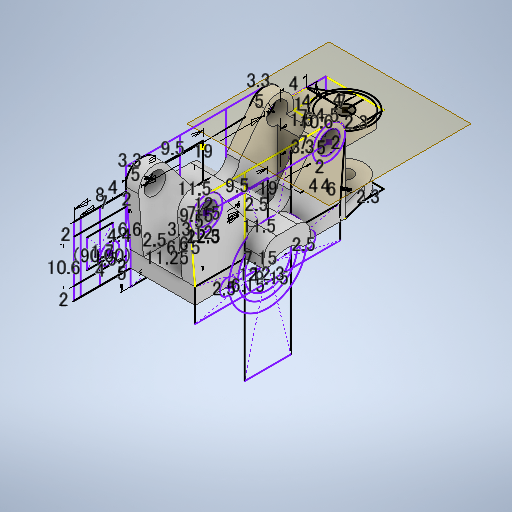
# Autodesk Inventor part: ikafly5.3d
Saved by Autodesk Inventor 2025 (Build 290162000, 162)
## iProperties
Created: 2024-06-20
Part Number: ikafly5.3d
Material: 一般
Document SubType Name: Modeling
Designer: Saigusa
Density: 1 g/cm^3
Appearance: 既定
Author: Saigusa
Autodesk Inventor part; units mm, degrees
ref_plane "YZ Plane" through (0, 0, 0) normal (1, 0, 0) x (0, 1, 0)
ref_plane "XZ Plane" through (0, 0, 0) normal (0, 1, 0) x (-1, 0, 0)
ref_plane "XY Plane" through (0, 0, 0) normal (0, 0, 1) x (1, 0, 0)
sketch "スケッチ1" plane through (0, 0, 0) normal (1, 0, 0) x (0, 1, 0)
  circle A0 centre (0, 0) radius 4.575
  circle A1 centre (0, 0) radius 3.575
  line L0 (0, 0) -> (0, 6)
  line L1 (0, 6) -> (0, -6)
  line L2 (0, 0) -> (11.5, 0)
  line L3 (11.5, 0) -> (11.5, 9.5)
  line L4 (11.5, 9.5) -> (11.5, -9.5)
  circle A2 centre (11.5, 9.5) radius 1.65
  circle A3 centre (11.5, -9.5) radius 1.65
  line L5 (0, 0) -> (0, 11.25)
  line L6 (0, 11.25) -> (0, -11.25)
  line L7 (-2.5, -11.25) -> (2.5, -11.25)
  line L8 (2.5, -11.25) -> (2.5, 11.25)
  line L9 (2.5, 11.25) -> (-2.5, 11.25)
  line L10 (-2.5, 11.25) -> (-2.5, -11.25)
  line L11 (-2.5, -11.25) -> (2.5, 11.25) construction
  line L12 (2.5, -11.25) -> (-2.5, 11.25) construction
  circle A4 centre (11.5, 9.5) radius 2.5
  circle A5 centre (11.5, -9.5) radius 2.5
  line L13 (2.5, 11.25) -> (11.2899, 11.9912)
  line L14 (2.5, -11.25) -> (11.2899, -11.9912)
  line L15 (14, 9.5) -> (14, -9.5)
  line L16 (0, -3.575) -> (14, -3.575)
  line L17 (0, 3.575) -> (14, 3.575)
  circle A6 centre (0, 0) radius 6
  line L18 (0, 0) -> (0, 6.15)
  line L19 (0, 6.15) -> (0, -6.15)
  circle A7 centre (0, 6.15) radius 1.25
  circle A8 centre (0, -6.15) radius 1.25
  line L20 (11.5, 9.5) -> (9, 9.5)
  line L21 (9, 9.5) -> (0, 9.5)
  line L22 (11.5, 9.5) -> (14, 9.5)
  line L23 (14, 9.5) -> (14, 11.9912)
  line L24 (14, 11.9912) -> (11.5, 11.9912)
  line L25 (11.5, 11.9912) -> (11.5, 9.5)
  line L26 (11.5, 11.9912) -> (0, 11.9912)
  line L27 (0, 11.9912) -> (0, 11.25)
  line L28 (0, 11.9912) -> (2, 11.9912)
  line L29 (2, 11.9912) -> (8.6, 11.9912)
  line L30 (8.6, 11.9912) -> (10.6, 11.9912)
  line L31 (0, 11.9912) -> (10.6, 11.9912)
  line L32 (10.6, 11.9912) -> (10.6, 19.9912)
  line L33 (10.6, 19.9912) -> (0, 19.9912)
  line L34 (0, 19.9912) -> (0, 11.9912)
  line L35 (0, 11.9912) -> (10.6, 11.9912)
  line L36 (10.6, 11.9912) -> (10.6, 15.9912)
  line L37 (10.6, 15.9912) -> (0, 15.9912)
  line L38 (0, 15.9912) -> (0, 11.9912)
  line L39 (0, 11.9912) -> (2, 11.9912)
  line L40 (2, 11.9912) -> (2, 19.9912)
  line L41 (2, 19.9912) -> (0, 19.9912)
  line L42 (0, 19.9912) -> (0, 11.9912)
  line L43 (10.6, 11.9912) -> (8.6, 11.9912)
  line L44 (8.6, 11.9912) -> (8.6, 19.9912)
  line L45 (8.6, 19.9912) -> (10.6, 19.9912)
  line L46 (10.6, 19.9912) -> (10.6, 11.9912)
  line L47 (0, 11.9912) -> (10.6, 11.9912)
  line L48 (10.6, 11.9912) -> (10.6, 18.9912)
  line L49 (10.6, 18.9912) -> (0, 18.9912)
  line L50 (0, 18.9912) -> (0, 11.9912)
  line L51 (0, 15.9912) -> (5.3, 15.9912)
  line L52 (7.5, 17.9912) -> (3.1, 17.9912)
  line L53 (3.1, 17.9912) -> (3.1, 13.9912)
  line L54 (3.1, 13.9912) -> (7.5, 13.9912)
  line L55 (7.5, 13.9912) -> (7.5, 17.9912)
  line L56 (7.5, 17.9912) -> (3.1, 13.9912) construction
  line L57 (3.1, 17.9912) -> (7.5, 13.9912) construction
  line L58 (5.3, 15.9912) -> (3.6, 15.9912)
  line L59 (3.6, 15.9912) -> (3.6, 14.4912)
  line L60 (3.6, 15.9912) -> (5.1, 15.9912) construction
  circle A9 centre (3.6, 14.4912) radius 0.5
  circle A10 centre (3.6, 14.4912) radius 1.5
  line L61 (5.1, 14.4912) -> (5.1, 11.9912)
  line L62 (11.5, -9.5) -> (0, -9.5)
  line L63 (0, -9.5) -> (0, -11.9912)
  line L64 (0, -11.9912) -> (11.5, -11.9912)
  line L65 (11.5, -11.9912) -> (11.5, -9.5)
  line L66 (0, -11.9912) -> (2, -11.9912)
  line L67 (2, -11.9912) -> (2, -18.9912)
  line L68 (2, -18.9912) -> (0, -18.9912)
  line L69 (0, -18.9912) -> (0, -11.9912)
  line L70 (0, -11.9912) -> (10.6, -11.9912)
  line L71 (10.6, -11.9912) -> (10.6, -15.9912)
  line L72 (10.6, -15.9912) -> (0, -15.9912)
  line L73 (0, -15.9912) -> (0, -11.9912)
  line L74 (10.6, -11.9912) -> (8.6, -11.9912)
  line L75 (8.6, -11.9912) -> (8.6, -18.9912)
  line L76 (8.6, -18.9912) -> (10.6, -18.9912)
  line L77 (10.6, -18.9912) -> (10.6, -11.9912)
  line L78 (2, -15.9912) -> (5.3, -15.9912)
  line L79 (3.05, -13.9912) -> (7.55, -13.9912)
  line L80 (7.55, -13.9912) -> (7.55, -17.9912)
  line L81 (7.55, -17.9912) -> (3.05, -17.9912)
  line L82 (3.05, -17.9912) -> (3.05, -13.9912)
  line L83 (3.05, -13.9912) -> (7.55, -17.9912) construction
  line L84 (7.55, -13.9912) -> (3.05, -17.9912) construction
  line L85 (5.3, -15.9912) -> (7, -15.9912)
  line L86 (7, -15.9912) -> (6.9874, -14.4912)
  circle A11 centre (6.9874, -14.4912) radius 0.5
  circle A12 centre (6.9874, -14.4912) radius 1.5
  line L87 (6.9874, -14.4912) -> (5.4874, -14.4912)
  line L88 (5.4874, -14.4912) -> (5.4874, -11.9912)
  line L89 (10.6, -11.9912) -> (10.6, -9.5)
  point P0 (0, 4.575)
  point P1 (0, -4.575)
  point P2 (2.5, 3.575)
  point P3 (2.5, 2.5555)
  point P4 (2.5, -2.5555)
  point P5 (2.5, -3.575)
  point P6 (0, 7.4)
  point P7 (0, 4.9)
  point P8 (0, -4.9)
  point P9 (0, -7.4)
  point P10 (2.5, 5.4544)
  point P11 (2.5, -5.4544)
  point P12 (4.8186, 3.575)
  point P13 (4.8186, -3.575)
  point P14 (2.8548, 3.575)
  point P15 (2.8548, -3.575)
  point P16 (9.85, 9.5)
  point P17 (11.5, 11.15)
  point P18 (11.5, -11.15)
  point P19 (9.85, -9.5)
  point P20 (5.5732, -13.9912)
  point P21 (6.9749, -15.9912)
  point P22 (8.6, -15.9912)
  point P23 (5.4874, -13.9912)
  point P24 (10.6, -10.8829)
  dimension "d0" = 9.15
  dimension "d1" = 7.15
  dimension "d2" = 6
  dimension "d3" = 12
  dimension "d6" = 11.5
  dimension "d7" = 9.5
  dimension "d8" = 19
  dimension "d9" = 3.3
  dimension "d10" = 3.3
  dimension "d11" = 11.25
  dimension "d12" = 22.5
  dimension "d13" = 5
  dimension "d14" = 5
  dimension "d15" = 5
  dimension "d28" = 12
  dimension "d29" = 6.15
  dimension "d30" = 12.3
  dimension "d31" = 2.5
  dimension "d32" = 2.5
  dimension "d99" = 2
  dimension "d100" = 6.6
  dimension "d101" = 2
  dimension "d114" = 10.6
  dimension "d115" = 8
  dimension "d116" = 4
  dimension "d117" = 2
  dimension "d118" = 2
  dimension "d119" = 7
  dimension "d120" = 4.4
  dimension "d121" = 4
  dimension "d122" = 1.7
  dimension "d123" = 1.5
  dimension "d124" = 90
  dimension "d125" = 2
  dimension "d126" = 7
  dimension "d127" = 10.6
  dimension "d128" = 4
  dimension "d129" = 7
  dimension "d130" = 4.5
  dimension "d131" = 4
  dimension "d132" = 1.5
  dimension "d133" = 1
  constraints: 180 end point, 27 parallel, 26 point on line, 21 perpendicular, 17 horizontal, 13 coincident, 12 centre point, 9 midpoint, 9 point on circle, 7 tangent, 2 vertical, 1 horizontal alignment, 2 other
  measures "d0" diameter of A0
  measures "d1" diameter of A1
  measures "d2" distance of L0.start L0.end
  measures "d3" distance of L0.end L1.end
  measures "d6" distance of L0.start L2.end
  measures "d7" distance of L2.end L3.end
  measures "d8" distance of L3.end L4.end
  measures "d9" diameter of A2
  measures "d10" diameter of A3
  measures "d11" distance of L0.start L5.end
  measures "d12" distance of L5.end L6.end
  measures "d13" distance of L9.end L8.end
  measures "d14" diameter of A4
  measures "d15" diameter of A5
  measures "d28" diameter of A6
  measures "d29" distance of L18.start L18.end
  measures "d30" distance of L18.end L19.end
  measures "d31" diameter of A7
  measures "d32" diameter of A8
  measures "d99" distance of L26.end L28.end
  measures "d100" distance of L28.end L29.end
  measures "d101" distance of L29.end L30.end
  measures "d114" distance of L33.end L32.end
  measures "d115" distance of L32.end L31.end
  measures "d116" distance of L36.end L35.end
  measures "d117" distance of L41.end L40.end
  measures "d118" distance of L44.end L45.end
  measures "d119" distance of L48.end L47.end
  measures "d120" distance of L54.end L53.end
  measures "d121" distance of L53.end L52.end
  measures "d122" distance of L51.end L58.end
  measures "d123" distance of L58.end L59.end
  measures "d124" angle of L59 L60
  measures "d125" distance of L67.end L68.end
  measures "d126" distance of L66.end L67.end
  measures "d127" distance of L71.end L72.end
  measures "d128" distance of L70.end L71.end
  measures "d129" distance of L75.end L74.end
  measures "d130" distance of L80.end L81.end
  measures "d131" distance of L79.end L80.end
  measures "d132" distance of L85.end L86.end
  measures "d133" diameter of A11
extrude "押し出し7" add sketch "スケッチ1" along normal blind 2 contours L2 A6 L16 A0 | A0 L17 A6 L2 | A0 L8 A6 L17 | L16 A6 L8 A0 | A6 L17 L3 L2 | L2 L4 L16 A6 | A0 L0 A7 A6 L8 | A6 L8 L21 A4 L3 L17 | L8 A6 A8 L1 A0 | L16 L4 A5 L62 L8 A6 | L3 L17 L15 L16 L4 | A6 A7 L5 L21 L8 | L3 A4 L15 L17 | L8 L62 L6 A8 A6 | L16 L15 A5 L4 | L21 L5 L9 L8 | L8 L13 A4 L21 | A4 L20 A2 L3 | L3 A2 L22 A4 | L62 A5 L89 L14 L8 | L8 L7 L6 L62 | A5 L64 L65 A3 L4 | L4 A3 L62 A5 | A4 L26 L25 A2 L20 | L22 A2 L25 L24 A4 | L62 A3 L89 A5 | A4 L24 L26 | L89 A5 L14 | L89 A3 L65 L64 A5
extrude "押し出し8" add sketch "スケッチ1" along normal blind 10 contours L2 A6 L16 A0 | A0 L17 A6 L2 | A0 L8 A6 L17 | L16 A6 L8 A0 | A6 L17 L3 L2 | L2 L4 L16 A6 | A0 L0 A7 A6 L8 | L8 A6 A8 L1 A0 | L3 L17 L15 L16 L4 | A6 A7 L5 L21 L8 | L8 L62 L6 A8 A6 | L0 A6 A7 | L21 L5 L9 L8 | A6 L5 A7 | A8 A6 L1 | L8 L7 L6 L62 | A8 L6 A6 picked at (0.2292, 5.6392) picked at (0.3961, 6.4211) picked at (0.2292, -5.6392) picked at (0.3961, -6.4211)
sketch "スケッチ6" plane through (10, 0, 0) normal (1, 0, 0) x (0, 0, -1)
  line L0 (0, 0) -> (-6.15, 0)
  line L1 (-6.15, 0) -> (6.15, 0)
  circle A0 centre (-6.15, 0) radius 1.25
  circle A1 centre (6.15, 0) radius 1.25
  line L2 (-11.25, 2.5) -> (11.25, 2.5)
  line L3 (11.25, 2.5) -> (11.25, -2.5)
  line L4 (11.25, -2.5) -> (-11.25, -2.5)
  line L5 (-11.25, -2.5) -> (-11.25, 2.5)
  line L6 (-11.25, 2.5) -> (11.25, -2.5) construction
  line L7 (11.25, 2.5) -> (-11.25, -2.5) construction
  line L8 (0, 0) -> (0, 11.5)
  line L9 (0, 11.5) -> (-9.5, 11.5)
  line L10 (-9.5, 11.5) -> (9.5, 11.5)
  circle A2 centre (-9.5, 11.5) radius 1.65
  circle A3 centre (-9.5, 11.5) radius 2.5
  circle A4 centre (9.5, 11.5) radius 1.65
  circle A5 centre (9.5, 11.5) radius 2.5
  circle A6 centre (0, 0) radius 6
  circle A7 centre (0, 0) radius 4.575
  arc A8 (11.9912, 11.2899) -> (9.5, 14) centre (9.5, 11.5) ccw projected
  line L11 (11.25, 2.5) -> (11.9912, 11.2899)
  line L12 (-11.9912, 11.2899) -> (-11.25, 2.5) projected
  line L13 (-11.25, 2.5) -> (-11.9912, 11.2899)
  line L14 (9.5, 14) -> (-9.5, 14) projected
  arc A9 (-9.5, 14) -> (-11.9912, 11.2899) centre (-9.5, 11.5) ccw projected
  line L15 (-9.5, 14) -> (9.5, 14)
  circle A10 centre (0, 0) radius 3.575
  line L16 (-3.575, 14) -> (-3.575, 4.8186) projected
  line L17 (3.575, -14) -> (-3.575, -14)
  line L18 (-3.575, -14) -> (-3.575, 14)
  line L19 (-3.575, 14) -> (3.575, 14)
  line L20 (3.575, 14) -> (3.575, -14)
  line L21 (3.575, -14) -> (-3.575, 14) construction
  line L22 (-3.575, -14) -> (3.575, 14) construction
  point P0 (-5.4544, 2.5)
  point P1 (5.4544, 2.5)
  point P2 (7, 11.5)
  point P3 (-7, 11.5)
  point P4 (-3.575, 11.5)
  point P5 (-3.575, 4.8186)
  point P6 (-3.575, 2.5)
  point P7 (-2.5555, 2.5)
  point P8 (2.5555, 2.5)
  point P9 (3.575, 2.5)
  point P10 (3.575, 11.5)
  dimension "d69" = 12
  dimension "d56" = 6.15
  dimension "d57" = 12.3
  dimension "d58" = 2.5
  dimension "d59" = 2.5
  dimension "d62" = 11.5
  dimension "d63" = 9.5
  dimension "d64" = 19
  dimension "d65" = 3.3
  dimension "d66" = 5
  dimension "d67" = 3.3
  dimension "d68" = 5
  dimension "d70" = 9.15
  dimension "d79" = 7.15
  constraints: 40 end point, 9 coincident, 8 centre point, 5 equal length, 4 horizontal, 4 midpoint, 3 perpendicular, 2 point on line, 2 tangent, 1 vertical, 2 other
  measures "d56" distance of L0.start L0.end
  measures "d57" distance of L0.end L1.end
  measures "d58" diameter of A0
  measures "d59" diameter of A1
  measures "d62" distance of L0.start L8.end
  measures "d63" distance of L8.end L9.end
  measures "d64" distance of L9.end L10.end
  measures "d65" diameter of A2
  measures "d66" diameter of A3
  measures "d67" diameter of A4
  measures "d68" diameter of A5
  measures "d70" diameter of A7
  measures "d79" diameter of A10
extrude "押し出し9" add sketch "スケッチ6" against normal blind 2 contours L2 L12 A3 L9 L16 A6 | L16 L9 L8 A6 | A6 L20 L10 A5 L11 L2 | A6 L8 L10 L20 | L16 L14 L20 L10 L9 | L9 A3 L14 L16 | L20 L14 A5 L10 | A3 | A5
extrude "押し出し10" add sketch "スケッチ1" against normal blind 0.5 contours L2 A6 L16 A0 | A0 L17 A6 L2 | A6 L17 L3 L2 | L2 L4 L16 A6 | L3 L17 L15 L16 L4
sketch "スケッチ7" plane through (-0.5, 0, 0) normal (-1, 0, 0) x (0, 0, 1)
  circle A0 centre (0, 0) radius 3.575
  line L0 (-9.5, 14) -> (9.5, 14) projected
  line L1 (-3.575, 14) -> (3.575, 14)
  circle A1 centre (0, 0) radius 4.575
  line L2 (-11.25, 0) -> (-11.25, 2.5) projected
  line L3 (11.25, -2.5) -> (-11.25, -2.5)
  line L4 (-11.25, -2.5) -> (-11.25, 2.5)
  line L5 (-11.25, 2.5) -> (11.25, 2.5)
  line L6 (11.25, 2.5) -> (11.25, -2.5)
  line L7 (11.25, -2.5) -> (-11.25, 2.5) construction
  line L8 (-11.25, -2.5) -> (11.25, 2.5) construction
  line L9 (-3.575, 14) -> (-3.575, 0)
  line L10 (3.575, 14) -> (3.575, 0)
  point P0 (-3.575, 2.5)
  point P1 (-2.5555, 2.5)
  point P2 (2.5555, 2.5)
  point P3 (3.575, 2.5)
  dimension "d75" = 7.15
  dimension "d76" = 5
  constraints: 18 end point, 2 centre point, 2 coincident, 2 midpoint, 2 parallel, 2 point on circle, 2 point on line, 2 tangent, 1 horizontal, 1 perpendicular
  measures "d75" diameter of A0
  measures "d76" distance of L3.end L2.end
extrude "押し出し11" add sketch "スケッチ7" along normal blind 3 contours A0 L5 L9 A1 L10 | A1 L9 L0 L10
extrude "押し出し12" add sketch "スケッチ6" along normal blind 3 contours L2 L18 A7 L8 A10 | A10 L8 A7 L20 L2 | L18 A6 L8 A7 | A7 L8 A6 L20 | L16 L9 L8 A6 | A6 L8 L10 L20 | L16 L14 L20 L10 L9
hole "穴1" at (0, 0, -6.15) at (0, 0, 6.15) direction (1, 0, 0) diameter 2.4 depth 3
sketch "スケッチ8" plane through (13, 0, 0) normal (1, 0, 0) x (0, 0, -1)
  line L0 (-3.575, 2.5) -> (-3.575, 14) projected
  line L1 (3.575, 14) -> (3.575, 2.5) projected
  line L2 (-3.575, 14) -> (3.575, 14)
  line L3 (3.575, 14) -> (3.575, 2.5)
  line L4 (3.575, 2.5) -> (-3.575, 2.5)
  line L5 (-3.575, 2.5) -> (-3.575, 14)
  circle A0 centre (0, 0) radius 6
  line L6 (-3.575, 14) -> (3.575, 14)
  line L7 (3.575, 14) -> (3.575, 6)
  line L8 (3.575, 6) -> (-3.575, 6)
  line L9 (-3.575, 6) -> (-3.575, 14)
  dimension "d89" = 12
  constraints: 16 end point, 4 parallel, 2 horizontal, 2 perpendicular, 1 centre point, 1 coincident, 1 point on line
  measures "d89" diameter of A0
extrude "押し出し13" cut sketch "スケッチ8" against normal blind 16.5 contours L0 L2 L1 L8
fillet "フィレット1" radius 2 10 edges at (11.5, 6, -3.575) (11.5, 6, 3.575) (9, 6, 3.575) (9, 6, -3.575) (5, 6, 3.575) (5, 6, -3.575) (1, 6, 3.575) (-1.75, 6, 3.575) (1, 6, -3.575) (-1.75, 6, -3.575)
sketch "スケッチ9" plane through (10, 0, 0) normal (1, 0, 0) x (0, 0, -1)
  arc A0 (2.5555, 2.5) -> (-2.5555, 2.5) centre (0, 0) ccw projected
  line L0 (0, 0) -> (0, 11.5)
  line L1 (0, 11.5) -> (-9.5, 11.5)
  circle A1 centre (9.5, 11.5) radius 1.65 projected
  line L2 (-9.5, 11.5) -> (9.5, 11.5)
  circle A2 centre (-9.5, 11.5) radius 2.5
  circle A3 centre (9.5, 11.5) radius 2.5
  arc A4 (-3.575, 8) -> (-1.575, 6) centre (-1.575, 8) ccw projected
  line L3 (-3.575, 8) -> (-7.5334, 13.0435)
  arc A5 (1.575, 6) -> (3.575, 8) centre (1.575, 8) ccw projected
  line L4 (3.575, 8) -> (7.5334, 13.0435)
  line L5 (9.5, 14) -> (3.575, 14) projected
  line L6 (-3.575, 8) -> (3.575, 8)
  line L7 (3.575, 8) -> (3.575, 14)
  line L8 (3.575, 14) -> (-3.575, 14)
  line L9 (-3.575, 14) -> (-3.575, 8)
  line L10 (-3.575, 8) -> (-9.5, 8)
  line L11 (-9.5, 8) -> (-9.5, 14)
  line L12 (-9.5, 14) -> (-3.575, 14)
  line L13 (-3.575, 14) -> (-3.575, 8)
  line L14 (3.575, 8) -> (9.5, 8)
  line L15 (9.5, 8) -> (9.5, 14)
  line L16 (9.5, 14) -> (3.575, 14)
  line L17 (3.575, 14) -> (3.575, 8)
  dimension "d93" = 11.5
  dimension "d94" = 9.5
  dimension "d95" = 5
  dimension "d96" = 5
  constraints: 34 end point, 6 parallel, 4 perpendicular, 3 horizontal, 3 point on circle, 2 centre point, 2 coincident, 2 tangent, 1 vertical
  measures "d93" distance of L0.start L0.end
  measures "d94" distance of L0.end L1.end
  measures "d95" diameter of A2
  measures "d96" diameter of A3
extrude "押し出し14" cut sketch "スケッチ9" against normal blind 16.5 contours L3 L1 L9 | L7 L2 L4 | L1 L3 A2 L12 L9 | L7 L5 A3 L4 L2
ref_plane "作業平面2" through (10, 14, -9.5) normal (0, 1, 0) x (-1, 0, 0)
extrude "押し出し16" add sketch "スケッチ1" along normal blind 10 contours L62 A5 L89 L14 L8 | L8 L7 L6 L62 | L14 L89 L64 L63 L7 | L62 A3 L89 A5
extrude "押し出し17" add sketch "スケッチ1" along normal blind 2 contours L75 L72 L80 A12 L79 L88 L64 | A12 L87 A11 L86 | L86 A11 L79 L80 A12 | A12 L80 L72 | L79 A12 L88 | A12 L80 L79 | L79 A11 L87 A12
extrude "押し出し18" add sketch "スケッチ1" along normal blind 9 contours L64 L67 L72 L69 | L71 L72 L75 L64 | L72 L67 L68 L69 | L77 L76 L75 L72
sketch "スケッチ11" plane through (0, 10.6, -11.9912) normal (0, 1, 0) x (1, 0, 0)
  line L0 (9, 0) -> (0, 0) projected
  line L1 (2, 4) -> (2, 0) projected
  line L2 (0, 0) -> (2, 0)
  line L3 (2, 0) -> (2, 4)
  line L4 (2, 4) -> (0, 4)
  line L5 (0, 4) -> (0, 0)
  line L6 (2, 4) -> (6, 4)
  circle A0 centre (6, 4) radius 1.15
  circle A1 centre (6, 4) radius 3.5
  circle A2 centre (6, 4) radius 4
  line L7 (6, 4) -> (6, 7)
  line L8 (0, 7) -> (9, 7) projected
  line L9 (4.85, 4) -> (4.85, 7)
  line L10 (4.85, 7) -> (0, 4)
  line L11 (0, -4.6412) -> (0, 7) projected
  line L12 (6, 4) -> (0, 4)
  line L13 (0, 4) -> (0, 7)
  line L14 (0, 7) -> (6, 7)
  line L15 (6, 7) -> (6, 4)
  line L16 (6, 4) -> (9, 4)
  line L17 (9, 4) -> (9, 7)
  line L18 (9, 7) -> (6, 7)
  line L19 (6, 7) -> (6, 4)
  point P0 (0, -11.9912)
  point P1 (9, 5.8028)
  point P2 (7.8028, 7)
  dimension "d141" = 2.3
  dimension "d140" = 4
  dimension "d142" = 7
  constraints: 32 end point, 7 parallel, 4 point on line, 3 coincident, 3 horizontal, 3 perpendicular, 2 horizontal alignment, 2 vertical, 1 centre point, 4 other
  measures "d140" distance of L1.start L6.end
  measures "d142" diameter of A1
extrude "押し出し19" cut sketch "スケッチ11" against normal blind 10.6 contours A0 L7 L6 | L6 L16 A0 | L7 A0 L16
extrude "押し出し20" cut sketch "スケッチ11" against normal blind 2 contours L11 L8 A2 L10 | A2 L8 A1 L10 | L17 A1 L8 A2 | A2 L8 L17 | A1 L8 L10
sketch "スケッチ12" plane through (0, 0, -4.575) normal (0, -1, 0) x (1, 0, 0)
  line L0 (2, -7.4162) -> (9, -7.4162) projected
  line L1 (0, -14.4162) -> (9, -14.4162) projected
  line L2 (9, -7.4162) -> (0, -7.4162)
  line L3 (0, -7.4162) -> (0, -14.4162)
  line L4 (0, -14.4162) -> (9, -14.4162)
  line L5 (9, -14.4162) -> (9, -7.4162)
  line L6 (0, -7.4162) -> (2, -7.4162)
  line L7 (2, -7.4162) -> (2, -11.4162)
  line L8 (2, -11.4162) -> (0, -11.4162)
  line L9 (0, -11.4162) -> (0, -7.4162)
  line L10 (2, -11.4162) -> (6, -11.4162)
  circle A0 centre (6, -11.4162) radius 1.15 projected
  circle A1 centre (6, -11.4162) radius 1.15
  circle A2 centre (6, -11.4162) radius 3
  line L11 (3, -11.4162) -> (9, -11.4162)
  line L12 (9, -11.4162) -> (9, -7.4162)
  line L13 (9, -7.4162) -> (3, -7.4162)
  line L14 (3, -7.4162) -> (3, -11.4162)
  line L15 (9, -7.4162) -> (10, -7.4162) projected
  line L16 (9, -7.4162) -> (10, -7.4162)
  line L17 (10, -7.4162) -> (9, -11.4162)
  point P0 (0, 4.575)
  point P1 (9, -11.4162)
  point P2 (6, -14.4162)
  point P3 (9, -14.4162)
  point P4 (3, -7.4162)
  point P5 (9, -11.4162)
  dimension "d151" = 6
  dimension "d147" = 2
  dimension "d148" = 4
  dimension "d149" = 4
  dimension "d150" = 2.3
  constraints: 30 end point, 7 equal length, 4 horizontal, 3 perpendicular, 2 coincident, 1 centre point, 1 point on line, 3 other
  measures "d147" distance of L7.end L8.end
  measures "d148" distance of L6.end L7.end
  measures "d149" distance of L7.end L10.end
  measures "d150" diameter of A1
extrude "押し出し21" cut sketch "スケッチ12" against normal blind 2 contours L7 L8 L3 L2 | L0 L14 L10 L7 | L10 A2 L1 L3 L8 | L5 L1 A2
extrude "押し出し22" add sketch "スケッチ12" against normal blind 2 contours L15 L17 L5
